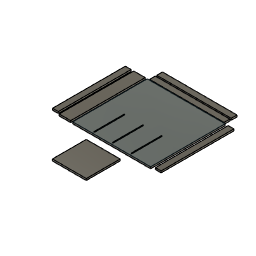
Robot Case v5 (Autodesk Fusion 360 design; units mm, degrees)
Autodesk Fusion 360 part; units mm, degrees
sketch "Sketch1" plane through (0, 0, 0) normal (0, 0, 1) x (1, 0, 0)
  line L0 (0, 0) -> (110, 0)
  line L1 (110, 0) -> (110, 110)
  line L2 (110, 110) -> (0, 110)
  line L3 (0, 110) -> (0, 0)
  dimension "d1" = 110
  dimension "d2" = 110
  constraint horizontal L0
  constraint vertical L1
  constraint horizontal L2
  constraint vertical L3
  constraint coincident L0.start L3.end
  measures "d1" distance of L0.start L0.end
  measures "d2" distance of L0.start L2.end
extrude "Extrude1" add sketch "Sketch1" along normal blind 2.5 makes body 1
sketch "Sketch2" plane through (0, 0, 0) normal (0, 0, 1) x (1, 0, 0)
  line L0 (-100, 0) -> (-50, 0)
  line L1 (-50, 0) -> (-50, 50)
  line L2 (-50, 50) -> (-100, 50)
  line L3 (-100, 50) -> (-100, 0)
  dimension "d5" = 50
  dimension "d6" = 50
  constraint horizontal L0
  constraint vertical L1
  constraint horizontal L2
  constraint vertical L3
  measures "d5" distance of L0.start L0.end
  measures "d6" distance of L0.start L2.end
extrude "Extrude2" add sketch "Sketch2" along normal blind 2.5 separate body makes body 2
move_body "Move1" bodies 2 to x (1, 0, 0) y (0, 1, 0) z (0, 0, 1) at (130, -50, 0)
sketch "Sketch3" plane through (0, 0, 2.5) normal (0, 0, 1) x (-1, 0, 0)
  line L0 (0, -110) -> (0, 0)
  line L1 (0, 0) -> (-110, 0)
  line L2 (-110, 0) -> (-110, -110)
  line L3 (-110, -110) -> (0, -110)
  line L4 (100, 40) -> (-10, 40)
  line L5 (-10, 40) -> (-10, 57)
  line L6 (-10, 57) -> (100, 57)
  line L7 (100, 57) -> (100, 40)
  dimension "d9" = 110
  dimension "d10" = 17
  constraint horizontal L4
  constraint vertical L5
  constraint horizontal L6
  constraint vertical L7
  measures "d9" distance of L4.start L4.end
  measures "d10" distance of L4.start L6.end
extrude "Extrude3" add sketch "Sketch3" along normal blind 2.5 separate body contours L4 L5 L6 L7 makes body 3
move_body "Move2" bodies 3 to x (1, 0, 0) y (0, 0, 1) z (0, -1, 0) at (0, -52, 62)
move_body "Move3" bodies 3 to x (1, 0, 0) y (0, 1, 0) z (0, 0, 1) at (100, 55, -2.5)
move_body "Move4" bodies 2 to x (1, 0, 0) y (0, 1, 0) z (0, 0, 1) at (0, 47, 19.5)
move_body "Move5" bodies 3 to x (1, 0, 0) y (0, 1, 0) z (0, 0, 1) at (0, 2, 0)
move_body "Move6" bodies 2 to x (1, 0, 0) y (0, 1, 0) z (0, 0, 1) at (0, -45, 0)
move_body "Move7" bodies 2 to x (1, 0, 0) y (0, 1, 0) z (0, 0, 1) at (0, 0.5, 0)
move_body "Move9" bodies 2 3 to x (1, 0, 0) y (0, 1, 0) z (0, 0, 1) at (0, -10, 0)
extrude "Extrude4" add 1 faces at (0, 73.3333, 1.6667) along direction (-1, 0, 0) blind 2.5 on bodies 1 bodies 1
extrude "Extrude5" add 1 faces at (110, 36.6667, 1.6667) along direction (1, 0, 0) blind 2.5 on bodies 1 bodies 1
sketch "Sketch4" plane through (0, 0, 0) normal (1, 0, 0) x (0, 1, 0)
sketch "Sketch5" plane through (0, 0, 2.5) normal (0, 0, 1) x (-1, 0, 0)
  line L0 (2.5, 0) -> (-112.5, 0)
  line L1 (-112.5, 0) -> (-112.5, -110)
  line L2 (-112.5, -110) -> (2.5, -110)
  line L3 (2.5, -110) -> (2.5, 0)
sketch "Sketch6" plane through (0, 0, 2.5) normal (0, 0, 1) x (-1, 0, 0)
  line L0 (10, 0) -> (18.5, 0)
  line L1 (18.5, 0) -> (18.5, -110)
  line L2 (18.5, -110) -> (10, -110)
  line L3 (10, -110) -> (10, 0)
  dimension "d34" = 8.5
  dimension "d35" = 110
  constraint horizontal L0
  constraint vertical L1
  constraint horizontal L2
  constraint vertical L3
  measures "d34" distance of L0.start L0.end
  measures "d35" distance of L0.start L2.end
extrude "Extrude6" add sketch "Sketch6" along normal blind 2.5 separate body makes body 4
copy_body "CopyPasteBodies2" bodies 4 makes body 5
move_body "Move10" bodies 5 to x (1, 0, 0) y (0, 1, 0) z (0, 0, 1) at (140, 0, 0)
move_body "Move11" bodies 4 to x (0, 0, -1) y (0, 1, 0) z (1, 0, 0) at (-15, 0, -5)
move_body "Move12" bodies 5 to x (0, 0, -1) y (0, 1, 0) z (1, 0, 0) at (125, 0, 135)
move_body "Move13" bodies 5 to x (1, 0, 0) y (0, 1, 0) z (0, 0, 1) at (-17.5, 0, -2.5)
move_body "Move14" bodies 4 to x (1, 0, 0) y (0, 1, 0) z (0, 0, 1) at (10, 0, -2.5)
extrude "Extrude7" cut 1 faces at (110.8333, 0, 5.3333) along direction (0, 1, 0) blind 2.5 on bodies 5 bodies 5
extrude "Extrude8" cut 1 faces at (-1.6667, 0, 5.3333) along direction (0, 1, 0) blind 2.5 on bodies 4 bodies 4
sketch "Sketch7" plane through (0, 0, 2.5) normal (0, 0, 1) x (-1, 0, 0)
  line L0 (-110, -113) -> (0, -113)
  line L1 (0, -113) -> (0, -115.5)
  line L2 (0, -115.5) -> (-110, -115.5)
  line L3 (-110, -115.5) -> (-110, -113)
  dimension "d50" = 110
  dimension "d51" = 2.5
  constraint horizontal L0
  constraint vertical L1
  constraint horizontal L2
  constraint vertical L3
  measures "d50" distance of L0.start L0.end
  measures "d51" distance of L0.start L2.end
extrude "Extrude9" add sketch "Sketch7" along normal blind 8.5 separate body makes body 6
move_body "Move15" bodies 6 to x (1, 0, 0) y (0, 1, 0) z (0, 0, 1) at (0, -5.5, 0)
sketch "Sketch8" plane through (0, 0, 0) normal (0, 0, 1) x (1, 0, 0)
  line L0 (-40, 15) -> (-39, 15)
  line L1 (-39, 15) -> (-39.5, 15.8636)
  line L2 (-39.5, 15.8636) -> (-40, 15)
  constraint horizontal L0
extrude "Extrude10" add sketch "Sketch8" along normal blind 45 separate body makes body 7
move_body "Move16" bodies 7 to x (1, 0, 0) y (0, 0, 1) z (0, -1, 0) at (0, 15, -15)
move_body "Move17" bodies 4 to x (1, 0, 0) y (0, 1, 0) z (0, 0, 1) at (-60, 0, 0)
move_body "Move18" bodies 7 to x (1, 0, 0) y (0, 1, 0) z (0, 0, 1) at (70, 32.5, 2.5)
move_body "Move19" bodies 7 to x (1, 0, 0) y (0, 1, 0) z (0, 0, 1) at (-30, 0, -30)
move_body "Move20" bodies 7 to x (1, 0, 0) y (0, 1, 0) z (0, 0, 1) at (0, 0, 30)
move_body "Move21" bodies 7 to x (1, 0, 0) y (0, 1, 0) z (0, 0, 1) at (0, -2.5, 0)
move_body "Move22" bodies 7 to x (1, 0, 0) y (0, 1, 0) z (0, 0, 1) at (0, 2.5, 0)
move_body "Move23" bodies 7 to x (1, 0, 0) y (0, 1, 0) z (0, 0, 1) at (-1.5, 0, 0)
move_body "Move24" bodies 7 to x (1, 0, 0) y (0, 1, 0) z (0, 0, 1) at (27.5, 0, 0)
copy_body "CopyPasteBodies3" bodies 7 makes body 8
move_body "Move25" bodies 8 to x (1, 0, 0) y (0, 1, 0) z (0, 0, 1) at (27.5, 0, 0)
copy_body "CopyPasteBodies4" bodies 8 makes body 9
move_body "Move26" bodies 9 to x (1, 0, 0) y (0, 1, 0) z (0, 0, 1) at (27.5, 0, 0)
move_body "Move27" bodies 5 to x (1, 0, 0) y (0, 1, 0) z (0, 0, 1) at (10, 0, 0)
copy_body "CopyPasteBodies5" bodies 6 makes body 10
move_body "Move28" bodies 10 to x (1, 0, 0) y (0, 1, 0) z (0, 0, 1) at (0, -60, 0)
move_body "Move29" bodies 4 to x (0, 0, 1) y (0, 1, 0) z (-1, 0, 0) at (-55.75, 0, 109.25)
move_body "Move30" bodies 5 to x (0, 0, -1) y (0, 1, 0) z (1, 0, 0) at (114.5, 0, 128)
move_body "Move31" bodies 2 to x (1, 0, 0) y (0, 1, 0) z (0, 0, 1) at (0, -5, -19.5)
move_body "Move32" bodies 3 to x (0, -1, 0) y (0, 0, -1) z (1, 0, 0) at (-41, 101.25, -7.75)
move_body "Move33" bodies 4 to x (1, 0, 0) y (0, 1, 0) z (0, 0, 1) at (0, 0, -46.75)
move_body "Move34" bodies 3 to x (1, 0, 0) y (0, 1, 0) z (0, 0, 1) at (0, 0, 0.25)
move_body "Move35" bodies 3 4 to x (1, 0, 0) y (0, 1, 0) z (0, 0, 1) at (16, 0, 0)
move_body "Move36" bodies 4 to x (1, 0, 0) y (0, 1, 0) z (0, 0, 1) at (16, 0, 0)
move_body "Move37" bodies 3 to x (1, 0, 0) y (0, 1, 0) z (0, 0, 1) at (0, 8.75, 0)
move_body "Move38" bodies 5 to x (1, 0, 0) y (0, 1, 0) z (0, 0, 1) at (0, 0, -5.5)
move_body "Move39" bodies 6 to x (1, 0, 0) y (0, 0, -1) z (0, 1, 0) at (0, 108.5, 110)
move_body "Move40" bodies 10 to x (1, 0, 0) y (0, 0, -1) z (0, 1, 0) at (0, 119, 50)
